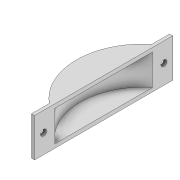
# Autodesk Inventor part: sprocket cover
Saved by Autodesk Inventor 2020 (Build 240168000, 168)
## iProperties
Created: 2020-02-13
Part Number: sprocket cover
Material: Generic
Document SubType Name: Modeling
Designer: ball
Density: 1 g/cm^3
Appearance: Default
Author: ball
Autodesk Inventor part; units mm, degrees
ref_plane "YZ Plane" through (0, 0, 0) normal (1, 0, 0) x (0, 1, 0)
ref_plane "XZ Plane" through (0, 0, 0) normal (0, 1, 0) x (-1, 0, 0)
ref_plane "XY Plane" through (0, 0, 0) normal (0, 0, 1) x (1, 0, 0)
sketch "Sketch1" plane through (0, 0, 0) normal (0, 1, 0) x (-1, 0, 0)
  circle A0 centre (-25.3492, 0) radius 35.56 construction
  line L0 (0, 84.1375) -> (6.35, 84.1375) construction
  line L1 (6.35, 84.1375) -> (6.35, -68.2625) construction
  line L2 (6.35, -68.2625) -> (0, -68.2625) construction
  line L3 (0, -68.2625) -> (0, 84.1375) construction
  arc A1 (0, -34.8078) -> (0, 34.8078) centre (-25.3492, 0) ccw
  line L4 (0, 34.8078) -> (0, -34.8078)
  point P0 (0, 0)
  point P1 (6.35, 29.1432)
  point P2 (6.35, -29.1432)
  dimension "d0" = 71.12
  dimension "d1" = 25.3492
  dimension "d2" = 6.35
  dimension "d3" = 152.4
  dimension "d4" = 86.12
  constraints: 10 end point, 4 point on circle, 4 point on line, 2 centre point, 2 parallel, 1 coincident, 1 collinear, 1 horizontal, 1 perpendicular
  measures "d0" diameter of A0
  measures "d1" distance of A0.centre point (0, 0)
  measures "d2" distance of L1.end L2.end
  measures "d3" distance of L0.end L1.end
  measures "d4" diameter of A1
extrude "Extrusion1" add sketch "Sketch1" along normal blind 25
shell "Shell2" thickness 2.5 removed faces 1 at (0, 8.3333, 11.6026)
sketch "Sketch2" plane through (0, 25, 0) normal (0, 1, 0) x (1, 0, 0)
  line L0 (0, 34.8078) -> (-2, 34.8078)
  line L1 (-2, 34.8078) -> (-2, 44.8078)
  line L2 (-2, 44.8078) -> (0, 44.8078)
  line L3 (0, 44.8078) -> (0, 34.8078)
  line L4 (-2, 34.8078) -> (0, 34.8078)
  line L5 (0.2807, 0) -> (-17.7108, 0) construction
  arc A0 (0, 34.8078) -> (0, -34.8078) centre (25.3492, 0) ccw construction
  line L6 (0, 34.8078) -> (-2, 34.8078)
  line L7 (-2, 34.8078) -> (-2, 33.2594)
  line L8 (-2, 33.2594) -> (0, 33.2594)
  line L9 (0, 33.2594) -> (0, 34.8078)
  line L10 (0, -34.8078) -> (-2, -34.8078)
  line L11 (-2, -34.8078) -> (-2, -44.8078)
  line L12 (-2, -44.8078) -> (0, -44.8078)
  line L13 (0, -44.8078) -> (0, -34.8078)
  line L14 (-2, -34.8078) -> (0, -34.8078)
  arc A1 (0, 34.8078) -> (0, -34.8078) centre (25.3492, 0) ccw construction
  line L15 (0, -34.8078) -> (-2, -34.8078)
  line L16 (-2, -34.8078) -> (-2, -33.2594)
  line L17 (-2, -33.2594) -> (0, -33.2594)
  line L18 (0, -33.2594) -> (0, -34.8078)
  point P0 (0, 0)
  dimension "d9" = 2
  dimension "d10" = 10
  dimension "d15" = 0
  dimension "d16" = 2
  constraints: 38 end point, 10 symmetric about line, 5 point on circle, 4 horizontal, 4 parallel, 2 perpendicular, 1 centre point, 1 other
  measures "d9" distance of L1.end L2.end
  measures "d10" distance of L0.end L1.end
  measures "d15" distance from line of L6.start L0
  measures "d16" distance of L8.end L7.end
extrude "Extrusion2" add sketch "Sketch2" against normal up to surface (25 mm away)
sketch "Sketch3" plane through (-2, 25, 33.2594) normal (-1, 0, 0) x (0, 0, 1)
  circle A0 centre (5.7742, -12.5) radius 1.9304
  line L0 (11.5484, -25) -> (0, -25) projected
  line L1 (0, 0) -> (11.5484, 0) projected
  line L2 (0, -25) -> (0, 0) projected
  line L3 (11.5484, 0) -> (11.5484, -25) projected
  circle A1 centre (-72.2929, -12.5) radius 1.9304
  line L4 (-78.0671, 0) -> (-78.0671, -25) projected
  line L5 (-78.0671, 0) -> (-66.5187, 0) projected
  point P0 (-33.2594, -25)
  dimension "d17" = 3.8608
  dimension "d18" = 25
  dimension "d19" = 12.5
  dimension "d20" = 11.5484
  dimension "d21" = 5.7742
  dimension "d22" = 3.8608
  dimension "d23" = 5.7742
  dimension "d24" = 12.5
  constraints: 2 centre point
  measures "d17" diameter of A0
  measures "d18" distance between parallel lines of L0 L1
  measures "d19" distance from line of L1 A0.centre
  measures "d20" distance between parallel lines of L2 L3
  measures "d21" distance from line of A0.centre L3
  measures "d22" diameter of A1
  measures "d23" distance from line of A1.centre L4
  measures "d24" distance from line of A1.centre L5
extrude "Extrusion3" cut sketch "Sketch3" against normal through all contours A0 | A1
equation "\"d19\" = 0.5 * d18"
equation "\"d21\" = 0.5 * d20"
equation "\"d23\" = d21"
equation "\"d24\" = d19"
body "Solid1"
